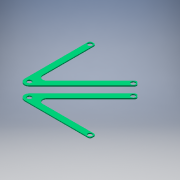
# Autodesk Inventor part: SolarFolds_Sketch
Saved by Autodesk Inventor 2016 (Build 200138000, 138)
## iProperties
Created: 2015-03-28
Part Number: SolarFolds_Sketch
Material: Generic
Document SubType Name: Modeling
Designer: Erin
Density: 1 g/cm^3
Appearance: Default
Author: Erin
Autodesk Inventor part; units mm, degrees
ref_plane "YZ Plane" through (0, 0, 0) normal (1, 0, 0) x (0, 1, 0)
ref_plane "XZ Plane" through (0, 0, 0) normal (0, 1, 0) x (-1, 0, 0)
sketch "Sketch1" plane through (0, 0, 0) normal (0, 0, 1) x (1, 0, 0)
  line L0 (-41.5, 58) -> (41.5, 58)
  line L1 (41.5, 58) -> (41.5, 158)
  line L2 (41.5, 158) -> (-41.5, 158)
  line L3 (-41.5, 158) -> (-41.5, 58)
  line L4 (58, 41.5) -> (158, 41.5)
  line L5 (158, 41.5) -> (158, -41.5)
  line L6 (158, -41.5) -> (58, -41.5)
  line L7 (58, -41.5) -> (58, 41.5)
  line L8 (-131.1952, 0) -> (204.4844, 0) construction
  line L9 (-48, 48) -> (48, 48)
  line L10 (48, 48) -> (48, -48)
  line L11 (48, -48) -> (-48, -48)
  line L12 (-48, -48) -> (-48, 48)
  line L13 (0, 180.9439) -> (0, -136.3054) construction
  point P0 (0, 0)
  point P1 (-48, 0)
  point P2 (0, 48)
  point P3 (0, 58)
  point P4 (58, 0)
  dimension "d0" = 83
  dimension "d1" = 100
  dimension "d2" = 100
  dimension "d3" = 83
  dimension "d5" = 96
  dimension "d6" = 96
  dimension "d7" = 10
  dimension "d8" = 10
  constraints: 28 end point, 7 parallel, 4 horizontal, 4 midpoint, 4 perpendicular, 2 horizontal alignment, 2 vertical alignment, 1 vertical
  measures "d0" distance of L2.end L1.end
  measures "d1" distance of L1.end L0.end
  measures "d2" distance of L5.end L6.end
  measures "d3" distance of L4.end L5.end
  measures "d5" distance of L9.start L9.end
  measures "d6" distance of L11.end L9.start
  measures "d7" distance between parallel lines of L9 L0
  measures "d8" distance between parallel lines of L7 L10
sketch "Sketch2" plane through (0, 0, 0) normal (0, 0, 1) x (1, 0, 0)
  line L0 (41.5, 158) -> (-41.5, 158) projected
  line L1 (41.5, 58) -> (41.5, 158) projected
  line L2 (-48, 48) -> (48, 48) projected
  line L3 (48, 48) -> (48, -48) projected
  line L4 (58, -41.5) -> (58, 41.5) projected
  line L5 (58, 41.5) -> (158, 41.5) projected
  line L6 (-41.5, 58) -> (41.5, 58) projected
  line L7 (158, 41.5) -> (158, -41.5) projected
  line L8 (48, 48) -> (136.7868, 136.7868) construction
  line L9 (35.5, 78) -> (57.5, 78)
  line L10 (57.5, 78) -> (57.5, 138)
  line L11 (57.5, 138) -> (35.5, 138)
  line L12 (35.5, 138) -> (35.5, 78)
  line L13 (41.5, 108) -> (-41.5, 108) construction
  line L14 (108, 41.5) -> (108, -41.5) construction
  line L15 (41.5, 158) -> (220.1006, 158) construction
  line L16 (158, 41.5) -> (158, 206.0131) construction
  line L17 (115.5736, 158) -> (158, 115.5736) construction
  line L18 (41.5, 138) -> (41.5, 78) construction
  line L19 (51.5, 138) -> (51.5, 78) construction
  line L20 (46.5, 138) -> (46.5, 78) construction
  line L21 (51.5, 158) -> (51.5, 70.6421)
  line L22 (60.0355, 67.1066) -> (133.2513, 140.3223)
  arc A0 (51.5, 158) -> (133.2513, 140.3223) centre (109.2071, 226.9991) ccw
  line L23 (68.9045, 84.4609) -> (84.4609, 68.9045)
  line L24 (84.4609, 68.9045) -> (126.8873, 111.331)
  line L25 (126.8873, 111.331) -> (111.331, 126.8873)
  line L26 (111.331, 126.8873) -> (68.9045, 84.4609)
  line L27 (80.2183, 73.1472) -> (122.6447, 115.5736) construction
  line L28 (105.6741, 90.1177) -> (90.1177, 105.6741) construction
  line L29 (73.1472, 80.2183) -> (115.5736, 122.6447) construction
  line L30 (76.6827, 76.6827) -> (119.1091, 119.1091) construction
  circle A1 centre (73.1472, 84.4609) radius 2.25
  circle A2 centre (111.331, 122.6447) radius 2.25
  circle A3 centre (84.4609, 73.1472) radius 2.25
  circle A4 centre (122.6447, 111.331) radius 2.25
  circle A5 centre (38.5, 135) radius 2.25
  circle A6 centre (38.5, 81) radius 2.25
  circle A7 centre (54.5, 135) radius 2.25
  circle A8 centre (54.5, 81) radius 2.25
  arc A9 (51.5, 70.6421) -> (60.0355, 67.1066) centre (56.5, 70.6421) ccw
  point P0 (0, 0)
  point P1 (158, 158)
  dimension "d23" = 30
  dimension "d25" = 45
  dimension "d30" = 10
  dimension "d37" = 10
  dimension "d38" = 60
  dimension "d39" = 4.5
  dimension "d40" = 3
  dimension "d42" = 4.5
  dimension "d43" = 3
  dimension "d46" = 60
  dimension "d47" = 30
  dimension "d48" = 4.5
  dimension "d49" = 3
  dimension "d50" = 3
  dimension "d51" = 4.5
  dimension "d52" = 3
  dimension "d53" = 3
  dimension "d54" = 5
  dimension "d55" = 25
  dimension "d57" = 3
  dimension "d58" = 3
  dimension "d59" = 3
  dimension "d60" = 3
  constraints: 46 end point, 15 perpendicular, 14 point on line, 10 centre point, 9 midpoint, 5 collinear, 4 point on circle, 4 symmetric about line, 3 parallel, 2 tangent, 1 horizontal, 4 other
  measures "d23" distance from line of point (158, 158) L17
  measures "d25" angle of L16 L17
  measures "d30" distance between parallel lines of L18 L19
  measures "d37" distance between parallel lines of L27 L29
  measures "d38" distance of L23.end L24.end
  measures "d39" diameter of A1
  measures "d40" distance from line of A1.centre L26
  measures "d42" diameter of A2
  measures "d43" distance from line of A2.centre L26
  measures "d46" distance of L9.end L10.end
  measures "d47" distance between parallel lines of L13 L11
  measures "d48" diameter of A5
  measures "d49" distance from line of A5.centre L11
  measures "d50" distance from line of A5.centre L12
  measures "d51" diameter of A6
  measures "d52" distance from line of A6.centre L9
  measures "d53" distance from line of A6.centre L12
  measures "d54" radius of A9
  measures "d55" distance between parallel lines of L17 L25
  measures "d57" distance from line of A5.centre L1
  measures "d58" distance from line of A7.centre L21
  measures "d59" distance from line of A4.centre L27
  measures "d60" distance from line of A2.centre L22
sketch "Sketch6" plane through (0, 0, 0) normal (0, 0, 1) x (1, 0, 0)
  line L0 (35.5, 78) -> (57.5, 78) projected
  circle A0 centre (54.5, 135) radius 2.25 projected
  line L1 (111.331, 126.8873) -> (68.9045, 84.4609) projected
  circle A1 centre (111.331, 122.6447) radius 2.25 projected
  line L2 (60.0355, 67.1066) -> (133.2513, 140.3223) projected
  arc A2 (51.5, 70.6421) -> (60.0355, 67.1066) centre (56.5, 70.6421) ccw projected
  line L3 (51.5, 158) -> (51.5, 70.6421) projected
  arc A3 (51.5, 158) -> (133.2513, 140.3223) centre (109.2071, 226.9991) ccw projected
  line L4 (119.1091, 119.1091) -> (76.6827, 76.6827) construction
  circle A4 centre (54.5, 135) radius 2.25
  circle A5 centre (111.331, 122.6447) radius 2.25
  circle A6 centre (56.5, 70.6421) radius 2.25
  line L5 (57.5, 138) -> (51.5, 138)
  line L6 (57.5, 138) -> (57.5, 83.3339)
  line L7 (111.331, 126.8873) -> (64.3853, 79.9416)
  line L8 (111.331, 126.8873) -> (115.5736, 122.6447)
  arc A7 (51.5, 70.6421) -> (60.0355, 67.1066) centre (56.5, 70.6421) ccw
  arc A8 (57.5, 83.3339) -> (64.3853, 79.9416) centre (61.7783, 83.3339) ccw
  line L9 (51.5, 138) -> (51.5, 70.6421)
  line L10 (115.5736, 122.6447) -> (60.0355, 67.1066)
  point P0 (0, 0)
  point P1 (38.5, 81)
  point P2 (38.5, 135)
  point P3 (126.8873, 111.331)
  point P4 (84.4609, 68.9045)
  dimension "d99" = 4.5
  constraints: 14 end point, 5 centre point, 5 tangent, 4 point on circle, 3 coincident, 2 collinear, 2 concentric, 2 point on line, 1 horizontal, 1 vertical
  measures "d99" diameter of A6
extrude "Extrusion13" add sketch "Sketch6" along normal blind 1 contours L8 L2 A2 L3 L5 L6 A8 L7 L1
fillet "Fillet1" radius 2 4 edges at (57.5, 138, 0.5) (51.5, 138, 0.5) (111.331, 126.8873, 0.5) (115.5736, 122.6447, 0.5)
ref_plane "Work Plane5" through (119.1091, 119.1091, 0) normal (-0.7071, 0.7071, 0) x (-0.7071, -0.7071, 0)
mirror "Mirror6" about plane through (119.1091, 119.1091, 0) normal (-0.7071, 0.7071, 0) of "Extrusion13", "Fillet1"
body "Solid2"
